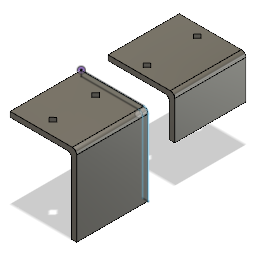
Head Magnet Mount (Autodesk Fusion 360 design; units mm, degrees)
Autodesk Fusion 360 part; units mm, degrees
sketch "Sketch1" plane through (0, 0, 0) normal (0, 0, 1) x (1, 0, 0)
  line L0 (0, 0) -> (34.9579, 0)
  line L1 (37.4579, -2.5) -> (37.4579, -45)
  line L2 (37.4579, -45) -> (34.4579, -45)
  line L3 (34.4579, -45) -> (34.4579, -5.25)
  line L4 (32.2079, -3) -> (0, -3)
  line L5 (0, -3) -> (0, 0)
  arc A0 (37.4579, -2.5) -> (34.9579, 0) centre (34.9579, -2.5) ccw
  arc A1 (34.4579, -5.25) -> (32.2079, -3) centre (32.2079, -5.25) ccw
  dimension "d3" = 45
  dimension "d5" = 3
  dimension "d6" = 3
  dimension "d30" = 2.5
  dimension "d31" = 2.25
  constraint horizontal L0
  constraint perpendicular L0 L1
  constraint perpendicular L1 L2
  constraint perpendicular L2 L3
  constraint perpendicular L1 L4
  constraint vertical L5
  constraint coincident L0.start L5.end
  constraint tangent L0 A0
  constraint tangent L1 A0
  constraint tangent L4 A1
  constraint tangent L3 A1
  measures "d3" distance of L0 L2
  measures "d5" distance of L0 L4
  measures "d6" distance of L1 L3
  measures "d30" radius of A0
  measures "d31" radius of A1
extrude "Extrude1" add sketch "Sketch1" along normal blind 40 makes body 1
sketch "Sketch2" plane through (0, -3, 0) normal (0, -1, 0) x (1, 0, 0)
  line L0 (0, 0) -> (32.2079, 0)
  line L1 (32.2079, 40) -> (0, 40)
  line L2 (0, 40) -> (0, 0)
  line L3 (16.104, 40) -> (16.104, -6.9864) construction
  circle A0 centre (16.104, 32) radius 2.2 construction
  circle A1 centre (16.104, 8) radius 2.2 construction
  line L4 (16.104, 34.2) -> (13.9042, 31.9656)
  line L5 (13.9042, 31.9656) -> (16.104, 29.8)
  line L6 (16.104, 29.8) -> (18.3037, 32.0344)
  line L7 (18.3037, 32.0344) -> (16.104, 34.2)
  line L8 (16.104, 10.2) -> (13.9042, 7.9656)
  line L9 (13.9042, 7.9656) -> (16.104, 5.8)
  line L10 (16.104, 5.8) -> (18.3037, 8.0344)
  line L11 (18.3037, 8.0344) -> (16.104, 10.2)
  line L12 (32.2079, 0) -> (32.2079, 40)
  dimension "d9" = 4.4
  dimension "d10" = 4.4
  dimension "d11" = 8
  dimension "d12" = 8
  constraint midpoint L1 L3.start
  constraint perpendicular L0 L3
  constraint coincident L3 A0.centre
  constraint coincident L3 A1.centre
  constraint coincident L3 L4.start
  constraint coincident A0 L4.start
  constraint coincident A0 L4.end
  constraint coincident A0 L5.end
  constraint coincident L3 L5.end
  constraint coincident A0 L6.end
  constraint perpendicular L5 L6
  constraint coincident A1 L8.start
  constraint coincident L3 L8.start
  constraint coincident A1 L8.end
  constraint perpendicular L7 L8
  constraint coincident A1 L9.end
  constraint coincident L3 L9.end
  constraint coincident A1 L10.end
  constraint perpendicular L9 L10
  measures "d9" diameter of A0
  measures "d10" diameter of A1
  measures "d11" distance of L3.start A0.centre
  measures "d12" distance of L0 A1.centre
extrude "Extrude2" cut sketch "Sketch2" against normal up to surface (3 mm away) contours L4 L5 L6 L7 | L8 L9 L10 L11 bodies 1
sketch "Sketch3" plane through (34.4579, 0, 0) normal (-1, 0, 0) x (0, 0, 1)
  line L0 (0, -5.25) -> (0, -45)
  line L1 (0, -45) -> (40, -45)
  line L2 (40, -45) -> (40, -5.25)
  line L3 (40, -25.125) -> (0, -25.125) construction
  line L4 (20, -18) -> (20, -57.3531) construction
  line L5 (12.7, -43.4) -> (30.8651, -43.4) construction
  line L6 (20, -7.3531) -> (29.1234, -7.3531) construction
  line L7 (20, -7.3531) -> (27.0476, -7.3531) construction
  line L8 (20, -7.3531) -> (23.8082, -7.3531) construction
  line L9 (5.3632, -9.0418) -> (35.3632, -9.0418)
  line L10 (35.3632, -9.0418) -> (35.3632, -40.7082)
  line L11 (35.3632, -40.7082) -> (5.3632, -40.7082)
  line L12 (5.3632, -40.7082) -> (5.3632, -9.0418)
  line L13 (40, -5.25) -> (0, -5.25)
  line L14 (20, -45) -> (20, 12.6333) construction
  line L15 (40, -45) -> (40, 32.8813) construction
  point P0 (80, -25.125)
  dimension "d27" = 30
  constraint midpoint L2 L3.start
  constraint midpoint L0 L3.end
  constraint perpendicular L1 L4
  constraint horizontal L6
  constraint horizontal L7
  constraint coincident L4 L6.start
  constraint horizontal L8
  constraint horizontal L9
  constraint vertical L10
  constraint horizontal L11
  constraint vertical L12
  constraint midpoint L1 L14.start
  constraint perpendicular L13 L14
  constraint coincident L4.end L14
  constraint coincident L1.end L2.start
  constraint perpendicular L1 L15
  constraint symmetric L3.end L15 P0
  measures "d27" distance of L10 L12
extrude "Extrude3" cut sketch "Sketch3" against normal blind 2.2 contours L9 L10 L11 L12 bodies 1
sketch "Sketch3 (2)" plane through (0, 0, 0) normal (0, 0, 1) x (1, 0, 0) in component "Mouth magnet mount"
  line L0 (0, 0) -> (34.9579, 0)
  line L1 (32.2079, -3) -> (0, -3)
  arc A0 (34.4579, -5.25) -> (32.2079, -3) centre (32.2079, -5.25) ccw
  arc A1 (37.4579, -2.5) -> (34.9579, 0) centre (34.9579, -2.5) ccw
  line L2 (0, -3) -> (0, 0)
  line L3 (31.9579, -3) -> (0, -3)
  line L4 (0, 0) -> (0, -3)
  line L5 (34.9579, 0) -> (0, 0)
  line L6 (34.4579, -5.5) -> (34.4579, -24.2562)
  line L7 (37.4579, -2.5) -> (37.4579, -24.2562)
  line L8 (37.4579, -24.2562) -> (34.4579, -24.2562)
  line L9 (34.9579, 0) -> (0, 0)
  line L10 (0, 0) -> (0, -3)
  line L11 (32.2079, -3) -> (0, -3)
  arc A2 (37.4579, -2.5) -> (34.9579, 0) centre (34.9579, -2.5) ccw
  arc A3 (34.4579, -5.5) -> (31.9579, -3) centre (31.9579, -5.5) ccw
  point P0 (34.9579, -2.5)
  point P1 (32.2079, -5.25)
  dimension "d37" = 2.5
  dimension "d38" = 2.5
  constraint coincident L1.end L2.start
  constraint coincident L0.start L2.end
  constraint coincident L0.end A1.end
  constraint tangent A0 L6
  constraint tangent A1 L7
  constraint horizontal L8
  constraint coincident L1.start A0.end
  constraint tangent L9 A2
  constraint tangent L7 A2
  constraint tangent L3 A3
  constraint tangent L6 A3
  constraint vertical L7
  measures "d37" radius of A2
  measures "d38" radius of A3
extrude "Extrude2'" add sketch "Sketch3 (2)" along normal blind 40 separate body makes body 2 in component "Mouth magnet mount"
move_body "Move1" bodies 2 to x (1, 0, 0) y (0, 1, 0) z (0, 0, 1) at (0, 0, -55) in component "Mouth magnet mount"
sketch "Sketch5" plane through (0, -3, 0) normal (0, -1, 0) x (1, 0, 0) in component "Mouth magnet mount"
  line L0 (0, -55) -> (31.9579, -55)
  line L1 (31.9579, -55) -> (31.9579, -15)
  line L2 (31.9579, -15) -> (0, -15)
  line L3 (0, -15) -> (0, -55)
  line L4 (15.979, -15) -> (15.979, -55) construction
  line L5 (15.979, -18.7574) -> (18.1003, -20.8787)
  line L6 (18.1003, -20.8787) -> (15.979, -23)
  line L7 (15.979, -23) -> (13.8576, -20.8787)
  line L8 (13.8576, -20.8787) -> (15.979, -18.7574)
  line L9 (13.924, -49.1299) -> (16.0366, -47)
  line L10 (16.0366, -47) -> (18.125, -49.1538)
  line L11 (18.125, -49.1538) -> (16.0383, -51.2352)
  line L12 (16.0383, -51.2352) -> (13.924, -49.1299)
  point P0 (15.979, -45)
  dimension "d41" = 3
  dimension "d42" = 3
  dimension "d43" = 3
  dimension "d44" = 3
  dimension "d45" = 8
  dimension "d46" = 8
  constraint midpoint L2 L4.start
  constraint midpoint L0 L4.end
  constraint coincident L4 L5.start
  measures "d41" distance of L5.start L5.end
  measures "d42" distance of L5.start L7.end
  measures "d43" distance of L9.end L10.end
  measures "d44" distance of L9.end L9.start
  measures "d45" distance of L2 L6.end
  measures "d46" distance of L0 L9.end
extrude "Extrude3'" cut sketch "Sketch5" against normal up to surface (3 mm away) contours L5 L6 L7 L8 | L9 L10 L11 L12 bodies 2 in component "Mouth magnet mount"
sketch "Sketch6" plane through (34.4579, 0, 0) normal (-1, 0, 0) x (0, 0, 1) in component "Mouth magnet mount"
  line L0 (-55, -5.5) -> (-55, -24.2562)
  line L1 (-55, -24.2562) -> (-15, -24.2562)
  line L2 (-15, -24.2562) -> (-15, -5.5)
  line L3 (-15, -5.5) -> (-55, -5.5)
  line L4 (-48.222, -7.4066) -> (-21.9025, -7.4066)
  line L5 (-21.9025, -7.4066) -> (-21.9025, -22.4066)
  line L6 (-21.9025, -22.4066) -> (-48.222, -22.4066)
  line L7 (-48.222, -22.4066) -> (-48.222, -7.4066)
  line L8 (-48.222, -14.9066) -> (-8.2676, -14.9066) construction
  line L9 (-48.222, -14.9066) -> (-61.4349, -14.9066) construction
  dimension "d53" = 15
  constraint horizontal L4
  constraint vertical L5
  constraint horizontal L6
  constraint vertical L7
  constraint midpoint L7 L8.start
  constraint perpendicular L2 L8
  constraint perpendicular L0 L9
  measures "d53" distance of L4 L6
extrude "Extrude4" cut sketch "Sketch6" against normal blind 2.2 contours L4 L5 L6 L7 bodies 2 in component "Mouth magnet mount"
component "Mouth magnet mount" placed x (1, 0, 0) y (0, 1, 0) z (0, 0, 1) at (0, 0, 0)
equation "d10 = d9"
equation "d12 = d11"
equation "d46 = d45"
named bodies: "Eyes Magnet Mount"
